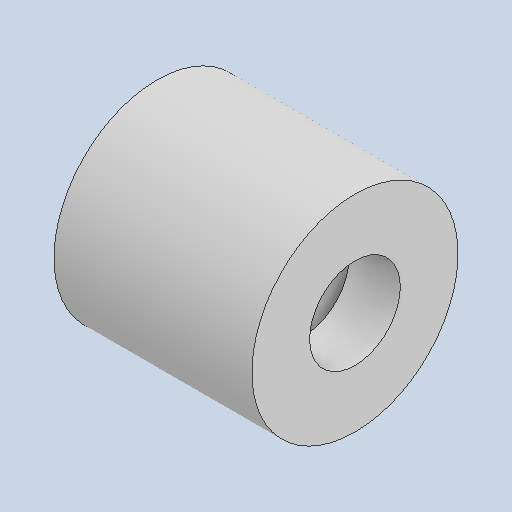
# Autodesk Inventor part: SpringCompensation_Outside_SupportPart_Zwischenstueck
Saved by Autodesk Inventor 2024 (Build 280153000, 153)
## iProperties
Created: 2022-10-13
Part Number: SpringCompensation_Outside_SupportPart_Zwischenstueck
Material: Generisch
Document SubType Name: Modeling
Designer: alexw
Density: 1 g/cm^3
Appearance: Vorgabe
Mass: 7.61286 g
Surface Area: 37.8562 cm^2
Volume: 7.61286 cm^3
Author: alexw
Autodesk Inventor part; units mm, degrees
ref_plane "YZ Plane" through (0, 0, 0) normal (1, 0, 0) x (0, 1, 0)
ref_plane "XZ Plane" through (0, 0, 0) normal (0, 1, 0) x (-1, 0, 0)
ref_plane "XY Plane" through (0, 0, 0) normal (0, 0, 1) x (1, 0, 0)
sketch "Skizze1" plane through (0, 0, 0) normal (0, 0, 1) x (1, 0, 0)
  line L0 (0, 0) -> (0, 12.5)
  line L1 (0, 12.5) -> (-24, 12.5)
  line L2 (-24, 12.5) -> (-24, 8)
  line L3 (-24, 8) -> (-6.2, 8)
  line L4 (-6.2, 8) -> (-6.2, 0)
  line L5 (-6.2, 0) -> (0, 0)
  line L6 (-16, 8) -> (-16, 0) construction
  line L7 (-6.2, 8.05) -> (-24, 8.05) construction
  dimension "d0" = 24
  dimension "d1" = 16
  dimension "d2" = 25
  dimension "d5" = 16.1
  dimension "d6" = 9.8
  dimension "d7" = 8
  constraints: 16 end point, 5 perpendicular, 4 point on line, 2 vertical, 1 horizontal
  measures "d0" distance between parallel lines of L0 L2
  measures "d1" diameter of L3 L5
  measures "d2" diameter of L1 L5
  measures "d5" diameter of L7 L5
  measures "d6" distance between parallel lines of L4 L6
  measures "d7" distance between parallel lines of L2 L6
revolve "Umdrehung1" add sketch "Skizze1" angle 360 about axis through (-6.2, 0, 0) along (1, 0, 0)
sketch "Skizze2" plane through (0, 0, 0) normal (1, 0, 0) x (0, 0, -1)
  point P0 (0, 0)
  point P1 (0, 0)
  constraints: 1 coincident
hole "Bohrung1" at (0, 0, 0) direction (-1, 0, 0) diameter 11 end through all clearance for "Inbusschraube DIN EN ISO 4762" size "M10" standard "DIN"
